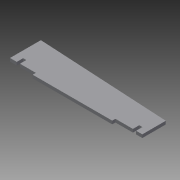
# Autodesk Inventor part: angle_plate_short_tall
Saved by Autodesk Inventor 2015 SP1 (Build 190203100, 203)
## iProperties
Created: 2016-08-03
Part Number: angle_plate_short_tall
Material: Generic
Document SubType Name: Modeling
Designer: polidorop
Density: 1 g/cm^3
Appearance: Default
Author: polidorop
Autodesk Inventor part; units mm, degrees
ref_plane "YZ Plane" through (0, 0, 0) normal (1, 0, 0) x (0, 1, 0)
ref_plane "XZ Plane" through (0, 0, 0) normal (0, 1, 0) x (-1, 0, 0)
ref_plane "XY Plane" through (0, 0, 0) normal (0, 0, 1) x (1, 0, 0)
sketch "Sketch1" plane through (0, 0, 0) normal (0, 0, 1) x (1, 0, 0)
  line L0 (-64, 50) -> (64, 50)
  line L1 (64, 50) -> (64, 0)
  line L2 (64, 0) -> (-64, 0)
  line L3 (-64, 0) -> (-64, 50)
  line L4 (-25, 0) -> (25, 0)
  line L5 (25, 0) -> (25, -2)
  line L6 (25, -2) -> (-25, -2)
  line L7 (-25, -2) -> (-25, 0)
  point P0 (0, 0)
  point P1 (0, 0)
  dimension "d0" = 50
  dimension "d1" = 128
  dimension "d2" = 2
  dimension "d3" = 50
  constraints: 16 end point, 4 parallel, 2 horizontal, 2 midpoint, 2 perpendicular, 1 coincident
  measures "d0" distance of L2.end L0.start
  measures "d1" distance of L0.start L0.end
  measures "d2" distance of L6.end L4.start
  measures "d3" distance of L5.end L6.end
extrude "Extrusion1" add sketch "Sketch1" along normal mid plane 2
sketch "Sketch2" plane through (0, 0, 1) normal (0, 0, 1) x (1, 0, 0)
  line L0 (-37.004, 19.1647) -> (37.8795, 15.001) projected
  line L1 (37.8795, 15.001) -> (37.8795, 6.0072) projected
  line L2 (37.8795, 6.0072) -> (-37.004, 10.1709) projected
  line L3 (-37.004, 10.1709) -> (-37.004, 19.1647) projected
  line L4 (-41.259, 17.7892) -> (-41.259, 8.0268) projected
  line L5 (41.9117, 3.4023) -> (41.9117, 13.1647) projected
  point P0 (0, 0)
sketch "Sketch3" plane through (0, 0, 1) normal (0, 0, 1) x (1, 0, 0)
  line L0 (-41.259, 17.7892) -> (-41.259, 8.0268) construction
  line L1 (-37.004, 19.1647) -> (37.8795, 15.001) construction
  line L2 (41.9117, 3.4023) -> (41.9117, 13.1647) construction
  line L3 (-41.259, 19.4013) -> (41.9117, 14.7768)
  line L4 (41.9117, 14.7768) -> (41.9117, 0)
  line L5 (91.9117, 0) -> (91.9117, 60)
  line L6 (91.9117, 60) -> (-91.259, 60)
  line L7 (-91.259, 60) -> (-91.259, 0)
  line L8 (-91.259, 0) -> (-41.259, 0)
  line L9 (-41.259, 0) -> (-41.259, 19.4013)
  line L10 (41.9117, 0) -> (91.9117, 0)
  point P0 (0, 0)
  dimension "d6" = 60
  dimension "d7" = 50
  dimension "d8" = 50
  constraints: 16 end point, 4 perpendicular, 4 point on line, 3 vertical, 1 collinear
  measures "d6" distance of L5.start L5.end
  measures "d7" distance of L4.end L5.start
  measures "d8" distance of L7.end L8.end
extrude "Extrusion2" cut sketch "Sketch3" against normal through all
sketch "Sketch4" plane through (0, 0, 1) normal (0, 0, 1) x (1, 0, 0)
  line L0 (36, 15.6306) -> (36, 0) projected
  line L1 (38, 15.6306) -> (36, 15.6306) projected
  line L2 (38, 0) -> (38, 15.6306) projected
  line L3 (36, 0) -> (38, 0) projected
  line L4 (-37, 19.7943) -> (-37, 0) projected
  line L5 (-35, 19.7943) -> (-37, 19.7943) projected
  line L6 (-35, 0) -> (-35, 19.7943) projected
  line L7 (-37, 0) -> (-35, 0) projected
  point P0 (0, 0)
sketch "Sketch5" plane through (0, 0, 1) normal (0, 0, 1) x (1, 0, 0)
  line L0 (-37, 19.7943) -> (-37, 0) construction
  line L1 (-35, 0) -> (-35, 19.7943) construction
  line L2 (36, 15.6306) -> (36, 0) construction
  line L3 (38, 0) -> (38, 15.6306) construction
  line L4 (-37, 4) -> (-35, 4)
  line L5 (-35, 4) -> (-35, 0)
  line L6 (-35, 0) -> (-37, 0)
  line L7 (-37, 0) -> (-37, 4)
  line L8 (38, 4) -> (36, 4)
  line L9 (36, 4) -> (36, 0)
  line L10 (36, 0) -> (38, 0)
  line L11 (38, 0) -> (38, 4)
  point P0 (0, 0)
  dimension "d11" = 4
  dimension "d12" = 4
  constraints: 16 end point, 4 parallel, 2 horizontal, 2 perpendicular, 2 point on line
  measures "d11" distance between parallel lines of L6 L4
  measures "d12" distance between parallel lines of L10 L8
extrude "Extrusion3" cut sketch "Sketch5" against normal through all
body "Solid1"
